Autodesk Inventor part; units mm, degrees
(part 5 of 6)
sketch "Block3" plane through (0, 0, 0) normal (0, 0, 1) x (1, 0, 0)
  arc A0 (-2.9788, 59.5057) -> (-3.9405, 59.975) centre (-5.1609, 56.2539) ccw
  arc A1 (-3.9405, 59.975) -> (-4.1922, 59.6845) centre (0, 56.3062) ccw
  arc A2 (-3.5908, 58.7994) -> (-3.7596, 58.5369) centre (0, 56.3062) ccw
  arc A3 (-3.7596, 58.5369) -> (-4.8145, 58.7162) centre (-4.9371, 54.802) ccw
  arc A4 (-4.8145, 58.7162) -> (-4.9742, 58.3666) centre (0, 56.3062) ccw
  arc A5 (-4.1478, 57.6868) -> (-4.2357, 57.3874) centre (0, 56.3062) ccw
  arc A6 (-4.9742, 58.3666) -> (-4.1478, 57.6868) centre (-2.0963, 61.0225) ccw
  arc A7 (-4.1922, 59.6845) -> (-3.5908, 58.7994) centre (-0.6827, 61.4221) ccw
  arc A8 (-4.1478, 54.9257) -> (-4.9742, 54.2459) centre (-2.0963, 51.59) ccw
  arc A9 (-4.9742, 54.2459) -> (-4.8145, 53.8963) centre (0, 56.3062) ccw
  arc A10 (-4.8145, 53.8963) -> (-3.7596, 54.0756) centre (-4.9371, 57.8105) ccw
  arc A11 (-3.7596, 54.0756) -> (-3.5908, 53.8131) centre (0, 56.3062) ccw
  arc A12 (-3.5908, 53.8131) -> (-4.1922, 52.928) centre (-0.6827, 51.1904) ccw
  arc A13 (-4.1922, 52.928) -> (-3.9405, 52.6375) centre (0, 56.3062) ccw
  arc A14 (-3.9405, 52.6375) -> (-2.9788, 53.1068) centre (-5.1609, 56.3586) ccw
  arc A15 (-2.9788, 53.1068) -> (-2.743, 52.9024) centre (0, 56.3062) ccw
  arc A16 (0.4673, 51.9598) -> (0.7762, 52.0042) centre (0, 56.3062) ccw
  arc A17 (0.1922, 50.9257) -> (0.4673, 51.9598) centre (-3.4193, 52.4401) ccw
  arc A18 (-0.1922, 50.9257) -> (0.1922, 50.9257) centre (0, 56.3062) ccw
  arc A19 (-0.4673, 51.9598) -> (-0.1922, 50.9257) centre (3.4193, 52.4401) ccw
  arc A20 (-0.7762, 52.0042) -> (-0.4673, 51.9598) centre (0, 56.3062) ccw
  arc A21 (-1.3315, 51.0895) -> (-0.7762, 52.0042) centre (-4.37, 53.5601) ccw
  arc A22 (-1.7003, 51.1978) -> (-1.3315, 51.0895) centre (0, 56.3062) ccw
  arc A23 (-1.6729, 52.2675) -> (-1.7003, 51.1978) centre (2.1915, 51.6334) ccw
  arc A24 (-1.9568, 52.3971) -> (-1.6729, 52.2675) centre (0, 56.3062) ccw
  arc A25 (-2.7473, 51.6759) -> (-1.9568, 52.3971) centre (-4.9666, 54.9025) ccw
  arc A26 (-2.743, 52.9024) -> (-3.0706, 51.8837) centre (0.7863, 51.2053) ccw
  arc A27 (-3.0706, 51.8837) -> (-2.7473, 51.6759) centre (0, 56.3062) ccw
  arc A28 (3.7596, 54.0756) -> (4.8145, 53.8963) centre (4.9371, 57.8105) ccw
  arc A29 (4.8145, 53.8963) -> (4.9742, 54.2459) centre (0, 56.3062) ccw
  arc A30 (4.9742, 54.2459) -> (4.1478, 54.9257) centre (2.0963, 51.59) ccw
  arc A31 (4.1478, 54.9257) -> (4.2357, 55.2251) centre (0, 56.3062) ccw
  arc A32 (4.2357, 55.2251) -> (5.2985, 55.3503) centre (4.3134, 59.1405) ccw
  arc A33 (5.2985, 55.3503) -> (5.3532, 55.7307) centre (0, 56.3062) ccw
  arc A34 (4.3687, 56.1502) -> (4.3687, 56.4623) centre (0, 56.3062) ccw
  arc A35 (5.3532, 55.7307) -> (4.3687, 56.1502) centre (3.3401, 52.3716) ccw
  arc A36 (4.3687, 56.4623) -> (5.3532, 56.8818) centre (3.3401, 60.2409) ccw
  arc A37 (5.2985, 57.2622) -> (4.2357, 57.3874) centre (4.3134, 53.472) ccw
  arc A38 (5.3532, 56.8818) -> (5.2985, 57.2622) centre (0, 56.3062) ccw
  arc A39 (3.0706, 60.7288) -> (2.7473, 60.9366) centre (0, 56.3062) ccw
  arc A40 (2.743, 59.7101) -> (3.0706, 60.7288) centre (-0.7863, 61.4072) ccw
  arc A41 (2.9788, 59.5057) -> (2.743, 59.7101) centre (0, 56.3062) ccw
  arc A42 (3.9405, 59.975) -> (2.9788, 59.5057) centre (5.1609, 56.2539) ccw
  arc A43 (4.1922, 59.6845) -> (3.9405, 59.975) centre (0, 56.3062) ccw
  arc A44 (3.7596, 58.5369) -> (3.5908, 58.7994) centre (0, 56.3062) ccw
  arc A45 (3.5908, 58.7994) -> (4.1922, 59.6845) centre (0.6827, 61.4221) ccw
  arc A46 (4.2357, 57.3874) -> (4.1478, 57.6868) centre (0, 56.3062) ccw
  arc A47 (4.9742, 58.3666) -> (4.8145, 58.7162) centre (0, 56.3062) ccw
  arc A48 (4.1478, 57.6868) -> (4.9742, 58.3666) centre (2.0963, 61.0225) ccw
  arc A49 (4.8145, 58.7162) -> (3.7596, 58.5369) centre (4.9371, 54.802) ccw
  arc A50 (-4.2357, 55.2251) -> (-4.1478, 54.9257) centre (0, 56.3062) ccw
  arc A51 (-5.2985, 55.3503) -> (-4.2357, 55.2251) centre (-4.3134, 59.1405) ccw
  arc A52 (-5.3532, 55.7307) -> (-5.2985, 55.3503) centre (0, 56.3062) ccw
  arc A53 (-4.3687, 56.4623) -> (-4.3687, 56.1502) centre (0, 56.3062) ccw
  arc A54 (-4.3687, 56.1502) -> (-5.3532, 55.7307) centre (-3.3401, 52.3716) ccw
  arc A55 (-5.2985, 57.2622) -> (-5.3532, 56.8818) centre (0, 56.3062) ccw
  arc A56 (-4.2357, 57.3874) -> (-5.2985, 57.2622) centre (-4.3134, 53.472) ccw
  arc A57 (-5.3532, 56.8818) -> (-4.3687, 56.4623) centre (-3.3401, 60.2409) ccw
  arc A58 (0.7762, 52.0042) -> (1.3315, 51.0895) centre (4.37, 53.5601) ccw
  arc A59 (1.3315, 51.0895) -> (1.7003, 51.1978) centre (0, 56.3062) ccw
  arc A60 (1.7003, 51.1978) -> (1.6729, 52.2675) centre (-2.1915, 51.6334) ccw
  arc A61 (2.7473, 60.9366) -> (1.9568, 60.2154) centre (4.9666, 57.71) ccw
  arc A62 (1.9568, 60.2154) -> (1.6729, 60.345) centre (0, 56.3062) ccw
  arc A63 (1.6729, 60.345) -> (1.7003, 61.4147) centre (-2.1915, 60.9791) ccw
  arc A64 (1.7003, 61.4147) -> (1.3315, 61.523) centre (0, 56.3062) ccw
  arc A65 (0.7762, 60.6083) -> (0.4673, 60.6527) centre (0, 56.3062) ccw
  arc A66 (1.3315, 61.523) -> (0.7762, 60.6083) centre (4.37, 59.0524) ccw
  arc A67 (-0.4673, 60.6527) -> (-0.7762, 60.6083) centre (0, 56.3062) ccw
  arc A68 (0.1922, 61.6868) -> (-0.1922, 61.6868) centre (0, 56.3062) ccw
  arc A69 (-0.1922, 61.6868) -> (-0.4673, 60.6527) centre (3.4193, 60.1724) ccw
  arc A70 (0.4673, 60.6527) -> (0.1922, 61.6868) centre (-3.4193, 60.1724) ccw
  arc A71 (3.5908, 53.8131) -> (3.7596, 54.0756) centre (0, 56.3062) ccw
  arc A72 (4.1922, 52.928) -> (3.5908, 53.8131) centre (0.6827, 51.1904) ccw
  arc A73 (3.9405, 52.6375) -> (4.1922, 52.928) centre (0, 56.3062) ccw
  arc A74 (2.9788, 53.1068) -> (3.9405, 52.6375) centre (5.1609, 56.3586) ccw
  arc A75 (2.743, 52.9024) -> (2.9788, 53.1068) centre (0, 56.3062) ccw
  arc A76 (1.6729, 52.2675) -> (1.9568, 52.3971) centre (0, 56.3062) ccw
  arc A77 (2.7473, 51.6759) -> (3.0706, 51.8837) centre (0, 56.3062) ccw
  arc A78 (1.9568, 52.3971) -> (2.7473, 51.6759) centre (4.9666, 54.9025) ccw
  arc A79 (3.0706, 51.8837) -> (2.743, 52.9024) centre (-0.7863, 51.2053) ccw
  arc A80 (-2.743, 59.7101) -> (-2.9788, 59.5057) centre (0, 56.3062) ccw
  arc A81 (-3.0706, 60.7288) -> (-2.743, 59.7101) centre (0.7863, 61.4072) ccw
  arc A82 (-2.7473, 60.9366) -> (-3.0706, 60.7288) centre (0, 56.3062) ccw
  arc A83 (-1.6729, 60.345) -> (-1.9568, 60.2154) centre (0, 56.3062) ccw
  arc A84 (-1.9568, 60.2154) -> (-2.7473, 60.9366) centre (-4.9666, 57.71) ccw
  arc A85 (-1.7003, 61.4147) -> (-1.6729, 60.345) centre (2.1915, 60.9791) ccw
  arc A86 (-0.7762, 60.6083) -> (-1.3315, 61.523) centre (-4.37, 59.0524) ccw
  arc A87 (-1.3315, 61.523) -> (-1.7003, 61.4147) centre (0, 56.3062) ccw
  point P0 (-0.0135, 56.3062)
  point P1 (-4.75, 56.3062)
sketch "Sketch1" plane through (0, 0, 0) normal (0, 0, 1) x (1, 0, 0)
  arc A0 (-1.2609, -14.9469) -> (-1.2609, 14.9469) centre (0, 0) ccw
  arc A1 (-8.2391, 14.9469) -> (-8.2391, -14.9469) centre (-9.5, 0) ccw
  line L0 (-9.5, 0) -> (0, 0) construction
  arc A2 (-8.2391, 14.9469) -> (-1.2609, 14.9469) centre (-4.75, 56.3062) ccw
  arc A3 (-1.2609, -14.9469) -> (-8.2391, -14.9469) centre (-4.75, -56.3062) ccw
  circle A4 centre (-4.75, 0) radius 11.5
  line L1 (-24.5, 15) -> (15, 15) construction
  line L2 (15, 15) -> (15, -15) construction
  line L3 (15, -15) -> (-24.5, -15) construction
  line L4 (-24.5, -15) -> (-24.5, 15) construction
  dimension "d0" = 9.5
  dimension "d2" = 15
  dimension "d4" = 23
  dimension "d13" = 39.5
  dimension "d14" = 0.2
  constraints: 10 end point, 8 point on circle, 8 tangent, 5 centre point, 2 equal radius, 2 horizontal, 2 parallel, 1 coincident, 1 midpoint, 1 perpendicular
  measures "d0" distance of L0.start L0.end
  measures "d2" radius of A1
  measures "d4" diameter of A4
  measures "d13" distance between parallel lines of L2 L4
  measures "d14" distance edge to line of A2 L1
extrude "Extrusion1" add sketch "Sketch1" along normal mid plane 11
sketch "Sketch8" plane through (0, 0, 5.5) normal (0, 0, 1) x (1, 0, 0)
  arc A0 (-1.2609, -14.9469) -> (-1.2609, 14.9469) centre (0, 0) ccw construction
  arc A1 (-8.2391, 14.9469) -> (-1.2609, 14.9469) centre (-4.75, 56.3062) ccw construction
  arc A2 (-8.2391, 14.9469) -> (-8.2391, -14.9469) centre (-9.5, 0) ccw construction
  arc A3 (-1.2609, -14.9469) -> (-8.2391, -14.9469) centre (-4.75, -56.3062) ccw construction
  circle A4 centre (-4.75, 0) radius 11.5 construction
  arc A5 (-1.2021, -14.2494) -> (-1.2021, 14.2494) centre (0, 0) ccw
  arc A6 (-1.2021, -14.2494) -> (-8.2979, -14.2494) centre (-4.75, -56.3062) ccw
  arc A7 (-8.2979, 14.2494) -> (-8.2979, -14.2494) centre (-9.5, 0) ccw
  arc A8 (-8.2979, 14.2494) -> (-1.2021, 14.2494) centre (-4.75, 56.3062) ccw
  dimension "d27" = 0.7
  constraints: 8 point on circle, 4 centre point, 3 other
  measures "d27" radial gap between concentric circles of A0 A5
extrude "Extrusion7" cut sketch "Sketch8" against normal blind 0.3
mirror "Mirror1" about plane through (0, 0, 0) normal (0, 0, 1) of "Extrusion7"
chamfer "Chamfer1" distance 0.3 angle 45 8 edges at (14.3, 0, 5.5) (-4.75, -14.1, 5.5) (-23.8, 0, 5.5) (-4.75, 14.1, 5.5) (14.3, 0, -5.5) (-4.75, 14.1, -5.5) (-23.8, 0, -5.5) (-4.75, -14.1, -5.5)
sketch "Sketch12" plane through (-4.75, -56.3062, -5.2) normal (0, 0, -1) x (-1, 0, 0)
  circle A0 centre (0, 56.3062) radius 11.5 projected
  circle A1 centre (0, 56.3062) radius 7.5
  point P0 (-4.75, 56.3062)
  dimension "d42" = 15
  constraints: 1 centre point, 1 coincident
  measures "d42" diameter of A1
extrude "Extrusion11" add sketch "Sketch12" along normal blind 5 and the other way blind 2.5 contours A1
spur gear teeth "Spur Gear1" teeth 24 pitch diameter 9.6 tip diameter 10.251 root diameter 8.451 face width 2 trims to tip circle yes start plane through (-4.75, 0, -10.2) normal (0, 0, -1) x (-1, 0, 0)
sketch "Sketch13" plane through (-4.75, 0, -8.2) normal (0, 0, -1) x (-1, 0, 0)
  arc A0 (2.4162, -4.5203) -> (2.7066, -4.3526) centre (0, 0) ccw projected
  arc A1 (1.7439, -3.8489) -> (2.4162, -4.5203) centre (4.6311, -1.6304) ccw projected
  arc A2 (1.4884, -3.9547) -> (1.7439, -3.8489) centre (0, 0) ccw projected
  arc A3 (1.4879, -4.9048) -> (1.4884, -3.9547) centre (-2.1219, -4.4276) ccw projected
  arc A4 (1.1639, -4.9916) -> (1.4879, -4.9048) centre (0, 0) ccw projected
  arc A5 (0.6883, -4.1691) -> (1.1639, -4.9916) centre (4.0514, -2.7734) ccw projected
  arc A6 (0.4142, -4.2052) -> (0.6883, -4.1691) centre (0, 0) ccw projected
  arc A7 (0.1677, -5.1228) -> (0.4142, -4.2052) centre (-3.1955, -3.7275) ccw projected
  arc A8 (-0.1677, -5.1228) -> (0.1677, -5.1228) centre (0, 0) ccw projected
  arc A9 (-0.4142, -4.2052) -> (-0.1677, -5.1228) centre (3.1955, -3.7275) ccw projected
  arc A10 (-0.6883, -4.1691) -> (-0.4142, -4.2052) centre (0, 0) ccw projected
  arc A11 (-1.1639, -4.9916) -> (-0.6883, -4.1691) centre (-4.0514, -2.7734) ccw projected
  arc A12 (-1.4879, -4.9048) -> (-1.1639, -4.9916) centre (0, 0) ccw projected
  arc A13 (-1.4884, -3.9547) -> (-1.4879, -4.9048) centre (2.1219, -4.4276) ccw projected
  arc A14 (-1.7439, -3.8489) -> (-1.4884, -3.9547) centre (0, 0) ccw projected
  arc A15 (-2.4162, -4.5203) -> (-1.7439, -3.8489) centre (-4.6311, -1.6304) ccw projected
  arc A16 (-2.7066, -4.3526) -> (-2.4162, -4.5203) centre (0, 0) ccw projected
  arc A17 (-2.4613, -3.4347) -> (-2.7066, -4.3526) centre (0.9036, -4.8259) ccw projected
  arc A18 (-2.6806, -3.2664) -> (-2.4613, -3.4347) centre (0, 0) ccw projected
  arc A19 (-3.5038, -3.7409) -> (-2.6806, -3.2664) centre (-4.8953, -0.3762) ccw projected
  arc A20 (-3.7409, -3.5038) -> (-3.5038, -3.7409) centre (0, 0) ccw projected
  arc A21 (-3.2664, -2.6806) -> (-3.7409, -3.5038) centre (-0.3762, -4.8953) ccw projected
  arc A22 (-3.4347, -2.4613) -> (-3.2664, -2.6806) centre (0, 0) ccw projected
  arc A23 (-4.3526, -2.7066) -> (-3.4347, -2.4613) centre (-4.8259, 0.9036) ccw projected
  arc A24 (-4.5203, -2.4162) -> (-4.3526, -2.7066) centre (0, 0) ccw projected
  arc A25 (-3.8489, -1.7439) -> (-4.5203, -2.4162) centre (-1.6304, -4.6311) ccw projected
  arc A26 (-3.9547, -1.4884) -> (-3.8489, -1.7439) centre (0, 0) ccw projected
  arc A27 (-4.9048, -1.4879) -> (-3.9547, -1.4884) centre (-4.4276, 2.1219) ccw projected
  arc A28 (-4.9916, -1.1639) -> (-4.9048, -1.4879) centre (0, 0) ccw projected
  arc A29 (-4.1691, -0.6883) -> (-4.9916, -1.1639) centre (-2.7734, -4.0514) ccw projected
  arc A30 (-4.2052, -0.4142) -> (-4.1691, -0.6883) centre (0, 0) ccw projected
  arc A31 (-5.1228, -0.1677) -> (-4.2052, -0.4142) centre (-3.7275, 3.1955) ccw projected
  arc A32 (-5.1228, 0.1677) -> (-5.1228, -0.1677) centre (0, 0) ccw projected
  arc A33 (-4.2052, 0.4142) -> (-5.1228, 0.1677) centre (-3.7275, -3.1955) ccw projected
  arc A34 (-4.1691, 0.6883) -> (-4.2052, 0.4142) centre (0, 0) ccw projected
  arc A35 (-4.9916, 1.1639) -> (-4.1691, 0.6883) centre (-2.7734, 4.0514) ccw projected
  arc A36 (-4.9048, 1.4879) -> (-4.9916, 1.1639) centre (0, 0) ccw projected
  arc A37 (-3.9547, 1.4884) -> (-4.9048, 1.4879) centre (-4.4276, -2.1219) ccw projected
  arc A38 (-3.8489, 1.7439) -> (-3.9547, 1.4884) centre (0, 0) ccw projected
  arc A39 (-4.5203, 2.4162) -> (-3.8489, 1.7439) centre (-1.6304, 4.6311) ccw projected
  arc A40 (-4.3526, 2.7066) -> (-4.5203, 2.4162) centre (0, 0) ccw projected
  arc A41 (-3.4347, 2.4613) -> (-4.3526, 2.7066) centre (-4.8259, -0.9036) ccw projected
  arc A42 (-3.2664, 2.6806) -> (-3.4347, 2.4613) centre (0, 0) ccw projected
  arc A43 (-3.7409, 3.5038) -> (-3.2664, 2.6806) centre (-0.3762, 4.8953) ccw projected
  arc A44 (-3.5038, 3.7409) -> (-3.7409, 3.5038) centre (0, 0) ccw projected
  arc A45 (-2.6806, 3.2664) -> (-3.5038, 3.7409) centre (-4.8953, 0.3762) ccw projected
  arc A46 (-2.4613, 3.4347) -> (-2.6806, 3.2664) centre (0, 0) ccw projected
  arc A47 (-2.7066, 4.3526) -> (-2.4613, 3.4347) centre (0.9036, 4.8259) ccw projected
  arc A48 (-2.4162, 4.5203) -> (-2.7066, 4.3526) centre (0, 0) ccw projected
  arc A49 (-1.7439, 3.8489) -> (-2.4162, 4.5203) centre (-4.6311, 1.6304) ccw projected
  arc A50 (-1.4884, 3.9547) -> (-1.7439, 3.8489) centre (0, 0) ccw projected
  arc A51 (-1.4879, 4.9048) -> (-1.4884, 3.9547) centre (2.1219, 4.4276) ccw projected
  arc A52 (-1.1639, 4.9916) -> (-1.4879, 4.9048) centre (0, 0) ccw projected
  arc A53 (-0.6883, 4.1691) -> (-1.1639, 4.9916) centre (-4.0514, 2.7734) ccw projected
  arc A54 (-0.4142, 4.2052) -> (-0.6883, 4.1691) centre (0, 0) ccw projected
  arc A55 (-0.1677, 5.1228) -> (-0.4142, 4.2052) centre (3.1955, 3.7275) ccw projected
  arc A56 (0.1677, 5.1228) -> (-0.1677, 5.1228) centre (0, 0) ccw projected
  arc A57 (0.4142, 4.2052) -> (0.1677, 5.1228) centre (-3.1955, 3.7275) ccw projected
  arc A58 (0.6883, 4.1691) -> (0.4142, 4.2052) centre (0, 0) ccw projected
  arc A59 (1.1639, 4.9916) -> (0.6883, 4.1691) centre (4.0514, 2.7734) ccw projected
  arc A60 (1.4879, 4.9048) -> (1.1639, 4.9916) centre (0, 0) ccw projected
  arc A61 (2.6806, -3.2664) -> (3.5038, -3.7409) centre (4.8953, -0.3762) ccw projected
  arc A62 (2.4613, -3.4347) -> (2.6806, -3.2664) centre (0, 0) ccw projected
  arc A63 (2.7066, -4.3526) -> (2.4613, -3.4347) centre (-0.9036, -4.8259) ccw projected
  circle A64 centre (0, 0) radius 7.5 projected
  arc A65 (3.9547, -1.4884) -> (4.9048, -1.4879) centre (4.4276, 2.1219) ccw projected
  arc A66 (3.8489, -1.7439) -> (3.9547, -1.4884) centre (0, 0) ccw projected
  arc A67 (4.5203, -2.4162) -> (3.8489, -1.7439) centre (1.6304, -4.6311) ccw projected
  arc A68 (4.3526, -2.7066) -> (4.5203, -2.4162) centre (0, 0) ccw projected
  arc A69 (3.4347, -2.4613) -> (4.3526, -2.7066) centre (4.8259, 0.9036) ccw projected
  arc A70 (3.2664, -2.6806) -> (3.4347, -2.4613) centre (0, 0) ccw projected
  arc A71 (3.7409, -3.5038) -> (3.2664, -2.6806) centre (0.3762, -4.8953) ccw projected
  arc A72 (3.5038, -3.7409) -> (3.7409, -3.5038) centre (0, 0) ccw projected
  arc A73 (2.7066, 4.3526) -> (2.4162, 4.5203) centre (0, 0) ccw projected
  arc A74 (2.4613, 3.4347) -> (2.7066, 4.3526) centre (-0.9036, 4.8259) ccw projected
  arc A75 (2.6806, 3.2664) -> (2.4613, 3.4347) centre (0, 0) ccw projected
  arc A76 (3.5038, 3.7409) -> (2.6806, 3.2664) centre (4.8953, 0.3762) ccw projected
  arc A77 (3.7409, 3.5038) -> (3.5038, 3.7409) centre (0, 0) ccw projected
  arc A78 (3.2664, 2.6806) -> (3.7409, 3.5038) centre (0.3762, 4.8953) ccw projected
  arc A79 (3.4347, 2.4613) -> (3.2664, 2.6806) centre (0, 0) ccw projected
  arc A80 (4.3526, 2.7066) -> (3.4347, 2.4613) centre (4.8259, -0.9036) ccw projected
  arc A81 (4.5203, 2.4162) -> (4.3526, 2.7066) centre (0, 0) ccw projected
  arc A82 (3.8489, 1.7439) -> (4.5203, 2.4162) centre (1.6304, 4.6311) ccw projected
  arc A83 (3.9547, 1.4884) -> (3.8489, 1.7439) centre (0, 0) ccw projected
  arc A84 (4.9048, 1.4879) -> (3.9547, 1.4884) centre (4.4276, -2.1219) ccw projected
  arc A85 (4.9916, 1.1639) -> (4.9048, 1.4879) centre (0, 0) ccw projected
  arc A86 (4.1691, 0.6883) -> (4.9916, 1.1639) centre (2.7734, 4.0514) ccw projected
  arc A87 (4.2052, 0.4142) -> (4.1691, 0.6883) centre (0, 0) ccw projected
  arc A88 (5.1228, 0.1677) -> (4.2052, 0.4142) centre (3.7275, -3.1955) ccw projected
  arc A89 (5.1228, -0.1677) -> (5.1228, 0.1677) centre (0, 0) ccw projected
  arc A90 (4.2052, -0.4142) -> (5.1228, -0.1677) centre (3.7275, 3.1955) ccw projected
  arc A91 (4.1691, -0.6883) -> (4.2052, -0.4142) centre (0, 0) ccw projected
  arc A92 (4.9916, -1.1639) -> (4.1691, -0.6883) centre (2.7734, -4.0514) ccw projected
  arc A93 (4.9048, -1.4879) -> (4.9916, -1.1639) centre (0, 0) ccw projected
  arc A94 (1.4884, 3.9547) -> (1.4879, 4.9048) centre (-2.1219, 4.4276) ccw projected
  arc A95 (1.7439, 3.8489) -> (1.4884, 3.9547) centre (0, 0) ccw projected
  arc A96 (2.4162, 4.5203) -> (1.7439, 3.8489) centre (4.6311, 1.6304) ccw projected
  point P0 (-4.75, 0)
extrude "Extrusion12" cut sketch "Sketch13" against normal through all
sketch "Sketch14" plane through (-4.75, -56.3062, -10.2) normal (0, 0, -1) x (-1, 0, 0)
  circle A0 centre (0, 56.3062) radius 11.5 projected
  circle A1 centre (0, 56.3062) radius 9.9126
  point P0 (-4.75, 56.3062)
  constraints: 1 centre point, 1 coincident
extrude "Extrusion13" cut sketch "Sketch14" against normal up to surface (5 mm away) contours A1
sketch "Sketch15" plane through (-1.5545, 3.7275, -5.2) normal (0, 0, -1) x (-0.9657677, 0.2594086, 0)
  circle A0 centre (2.1192, -4.4288) radius 11.5 projected
  circle A1 centre (2.1192, -4.4288) radius 3.95
  point P0 (-2.4682, -3.1967)
  dimension "d51" = 7.9
  constraints: 1 centre point, 1 coincident
  measures "d51" diameter of A1
extrude "Extrusion14" cut sketch "Sketch15" against normal through all contours A1
sketch "Sketch16" plane through (-4.75, 0, -5.2) normal (0, 0, -1) x (-0.9659258, -0.258819, 0)
  circle A0 centre (0, 0) radius 11.5 projected
  circle A1 centre (0, 0) radius 4.3255
  arc A2 (-3.2664, -2.6806) -> (-3.7409, -3.5038) centre (-0.3762, -4.8953) ccw projected
  circle A3 centre (0, 0) radius 4.2255
  point P0 (-4.5881, -1.2294)
  dimension "d54" = 0.1
  constraints: 2 coincident, 1 centre point, 3 other
extrude "Extrusion15" add sketch "Sketch16" against normal up to surface (2.5 mm away) contours A1
chamfer "Chamfer2" distance 2 distance2 1 1 edges at (-16.25, 0, -5.2) measured on face at (-16.25, 0, -4.7)
sketch "Sketch17" plane through (-4.75, -56.3062, -2.7) normal (0, 0, 1) x (1, 0, 0)
  circle A0 centre (0, 56.3062) radius 11.5 projected
  circle A1 centre (0, 56.3062) radius 3.95 projected
extrude "Extrusion16" add sketch "Sketch17" along normal blind 1.2
sketch "Sketch19" plane through (0, 0, 5.2) normal (0, 0, 1) x (1, 0, 0)
  circle A0 centre (-4.75, 0) radius 11.5 construction
  circle A1 centre (-4.75, 0) radius 13
  point P0 (0, 0)
  dimension "d67" = 26
  constraints: 1 centre point, 1 coincident
  measures "d67" diameter of A1
extrude "Extrusion17" cut sketch "Sketch19" against normal up to surface (6.7 mm away)
sketch "Sketch18" plane through (0, 0, 0) normal (0, 1, 0) x (-1, 0, 0)
  line L0 (4.75, -1.5) -> (4.75, 10.534) construction
  line L1 (17.75, 5.2) -> (13.3, 5.2)
  line L2 (13.8, 4.7) -> (13.8, 0.4)
  line L3 (13.8, 0.4) -> (13.3, 0.4)
  line L4 (13.3, 0.4) -> (13.3, -1.5)
  line L5 (13.3, -1.5) -> (4.75, -1.5) construction
  line L6 (-6.75, -1.5) -> (16.25, -1.5) construction
  line L7 (13.3, -1.5) -> (16.25, -1.5)
  line L8 (16.25, 5.2) -> (-6.75, 5.2) construction
  line L9 (-8.25, 5.2) -> (17.75, 5.2) construction
  line L10 (17.75, -1.5) -> (17.75, -1.5) construction
  line L11 (17.75, 5.2) -> (17.75, -1.5)
  line L12 (17.75, -1.5) -> (16.25, -1.5)
  line L13 (13.3, 5.2) -> (13.3, 4.7)
  line L14 (13.3, 4.7) -> (13.8, 4.7)
  point P0 (4.75, 5.2)
  dimension "d62" = 9.05
  dimension "d63" = 0.5
  dimension "d64" = 4.3
  dimension "d66" = 1.9
  dimension "d70" = 0
  dimension "d106" = 0.5
  dimension "d107" = 0.5
  constraints: 22 end point, 6 perpendicular, 3 vertical, 2 horizontal, 2 midpoint, 1 point on line
  measures "d62" distance between parallel lines of L0 L2
  measures "d63" distance of L2.end L3.end
  measures "d64" distance of L2.start L2.end
  measures "d66" distance of L3.end L4.end
  measures "d70" distance between parallel lines of L1 L9
  measures "d106" distance of L1.end L13.end
  measures "d107" distance of L13.end L2.start
revolve "Revolution1" add sketch "Sketch18" angle 360 about axis through (-4.75, 0, -1.5) along (0, 0, 1)
ref_plane "Work Plane2" through (0, 0, 0) normal (0, 0, 1) x (1, 0, 0)
sketch "Sketch21" plane through (0, 0, 0) normal (0, 0, 1) x (1, 0, 0)
  circle A0 centre (-4.75, 0) radius 9.05 projected
  line L0 (-4.75, 0) -> (-15.2041, 13.8731) construction
  line L1 (-4.75, 0) -> (-26.3613, 0) construction
  arc A1 (-8.2391, 14.9469) -> (-8.2391, -14.9469) centre (-9.5, 0) ccw construction
  line L2 (-15.2041, 13.8731) -> (-16.4078, 15.4704) construction
  line L3 (-16.4078, 15.4704) -> (-10.7682, 7.9864) construction
  line L4 (-15.2789, 12.7261) -> (-17.0067, 15.019)
  line L5 (-17.0067, 15.019) -> (-15.8088, 15.9217)
  line L6 (-15.8088, 15.9217) -> (-14.081, 13.6288)
  line L7 (-14.081, 13.6288) -> (-15.2789, 12.7261)
  line L8 (-15.2789, 12.7261) -> (-15.8088, 15.9217) construction
  line L9 (-17.0067, 15.019) -> (-14.081, 13.6288) construction
  point P0 (0, 0)
  point P1 (-13.588, 11.7284)
  point P2 (-15.5439, 14.3239)
  dimension "d75" = 53
  dimension "d76" = 2
  dimension "d81" = 16.5
  dimension "d82" = 1.5
  constraints: 22 end point, 4 midpoint, 3 parallel, 2 point on line, 1 collinear, 1 horizontal, 1 perpendicular, 1 point on circle
  measures "d75" angle of L0 L1
  measures "d76" distance of L0.end L2.end
  measures "d81" distance from line of L0.start L7
  measures "d82" distance of L4.end L5.end
extrude "Extrusion19" cut sketch "Sketch21" against normal mid plane 6 contours L4 L5 L6 L7
ref_plane "Work Plane3" through (-12.1194, 8.5333, 3) normal (-0.601815, 0.7986355, 0) x (0.7986355, 0.601815, 0)
sketch "Sketch24" plane through (-12.1194, 8.5333, 3) normal (-0.601815, 0.7986355, 0) x (0.7986355, 0.601815, 0)
  line L0 (0, 6) -> (0, 0) construction
  line L1 (0, 0) -> (1.5, 0) construction
  line L2 (1.5, 0) -> (1.5, 6) construction
  line L3 (1.5, 6) -> (0, 6) construction
  line L4 (-1.25, 7.75) -> (2.75, 7.75)
  line L5 (2.75, 7.75) -> (2.75, 6.25)
  line L6 (2.75, 6.25) -> (-1.25, 6.25)
  line L7 (-1.25, 6.25) -> (-1.25, 7.75)
  line L8 (-1.25, 7.75) -> (2.75, 6.25) construction
  line L9 (2.75, 7.75) -> (-1.25, 6.25) construction
  line L10 (0.75, 7) -> (0.75, 6) construction
  point P0 (4.5435, 3)
  dimension "d99" = 1
  dimension "d100" = 1.5
  dimension "d101" = 4
  constraints: 14 end point, 3 midpoint, 2 parallel, 1 horizontal, 1 perpendicular, 1 vertical
  measures "d99" distance of L10.start L10.end
  measures "d100" distance of L4.end L5.end
  measures "d101" distance of L4.start L4.end
sketch "Sketch25" plane through (-15.2789, 12.7261, 3) normal (-0.601815, 0.7986355, 0) x (0.7986355, 0.601815, 0)
  line L0 (0, 6) -> (0, 0) projected
  line L1 (0, 0) -> (1.5, 0) projected
  line L2 (1.5, 0) -> (1.5, 6) projected
  line L3 (1.5, 6) -> (0, 6) projected
  point P0 (4.5435, 3)
loft "Loft1" cut profiles "Sketch24", "Sketch25"
sketch "Sketch22" plane through (-4.75, 0, 5.2) normal (0, 0, 1) x (1, 0, 0)
  circle A0 centre (-9.5, -5.5) radius 1
  circle A1 centre (0, 0) radius 3.95 projected
  point P0 (4.75, 0)
  dimension "d88" = 5.5
  dimension "d89" = 9.5
  dimension "d90" = 2
  constraints: 1 centre point
  measures "d88" vertical distance of A0.centre A1.centre
  measures "d89" horizontal distance of A1.centre A0.centre
  measures "d90" diameter of A0
extrude "Extrusion20" cut sketch "Sketch22" against normal blind 4 contours A0
sketch "Sketch23" plane through (-14.25, -5.5, 1.2) normal (0, 0, 1) x (1, 0, 0)
  circle A0 centre (0, 0) radius 1 construction
  line L0 (0, 0) -> (-6.6144, -4.5) construction
  line L1 (-0.5625, 0.8268) -> (-7.1769, -3.6732)
  line L2 (-6.0519, -5.3268) -> (0.5625, -0.8268)
  arc A1 (0.5625, -0.8268) -> (-0.5625, 0.8268) centre (0, 0) ccw
  arc A2 (-7.1769, -3.6732) -> (-6.0519, -5.3268) centre (-6.6144, -4.5) ccw
  circle A3 centre (9.5, 5.5) radius 3.95 projected
  point P0 (-3.3072, -2.25)
  dimension "d93" = 10
  dimension "d94" = 8
  constraints: 8 end point, 4 point on circle, 4 tangent, 2 centre point, 1 concentric, 1 midpoint, 1 parallel
  measures "d93" vertical distance of A3.centre L0.end
  measures "d94" distance of L0.start L0.end
extrude "Extrusion21" cut sketch "Sketch23" along normal mid plane 3 contours A1 L2 A2 L1
pattern_circular "Circular Pattern2" count 2 over 360 about axis through (-4.75, 0, -5.2) along (0, 0, 1) of "Extrusion19", "Extrusion20", "Extrusion21", "Loft1"
fillet "Fillet2" radius 1 8 edges at (-20.7468, -9.9252, -0.3) (-21.3883, -9.147, 1.2) (-20.7468, -9.9252, 2.7) (-20.0545, -10.6585, 1.2) (11.2468, 9.9252, 2.7) (11.8883, 9.147, 1.2) (11.2468, 9.9252, -0.3) (10.5545, 10.6585, 1.2)
sketch "Sketch26" plane through (-4.75, -56.3062, -2.7) normal (0, 0, -1) x (-1, 0, 0)
  arc A0 (-5.2349, 46.0668) -> (8.3998, 64.1608) centre (0, 56.3062) ccw projected
  circle A1 centre (0, 56.3062) radius 11.45
  circle A2 centre (0, 56.3062) radius 23.5644
  arc A3 (-5.2349, 46.0668) -> (8.3998, 64.1608) centre (0, 56.3062) ccw projected
  circle A4 centre (0, 56.3062) radius 11.5
  point P0 (-4.75, 56.3062)
  point P1 (8.3998, 64.1608)
  dimension "d108" = 0.05
  constraints: 3 coincident, 2 centre point, 3 other
  measures "d108" radial gap between concentric circles of A0 A1
extrude "Extrusion22" cut sketch "Sketch26" along normal mid plane 36.5 contours A4 A0 | A2
ref_plane "Work Plane4" through (-4.75, -56.3062, -0.9) normal (0, 0, -1) x (-1, 0, 0)
sketch "Sketch27" plane through (-4.75, -56.3062, -0.9) normal (0, 0, -1) x (-1, 0, 0)
  circle A0 centre (0.0119, 55.9035) radius 37.3016
  point P0 (-4.75, 56.3062)
  constraints: 1 centre point
extrude "Extrusion23" cut sketch "Sketch27" against normal through all
sketch "Sketch28" plane through (-4.75, 0, -0.9) normal (0, 0, 1) x (1, 0, 0)
  line L0 (18.7681, 21.7252) -> (10, 21.7252)
  line L1 (10, 21.7252) -> (10, -19.8553)
  line L2 (10, -19.8553) -> (18.7681, -19.8553)
  line L3 (18.7681, -19.8553) -> (18.7681, 21.7252)
  line L4 (-19.6954, 20.4967) -> (-10, 20.4967)
  line L5 (-10, 20.4967) -> (-10, -19.0939)
  line L6 (-10, -19.0939) -> (-19.6954, -19.0939)
  line L7 (-19.6954, -19.0939) -> (-19.6954, 20.4967)
  circle A0 centre (0, 0) radius 3.95 projected
  line L8 (0, 0) -> (0, 16.0604) construction
  point P0 (4.75, 0)
  dimension "d116" = 10
  dimension "d117" = 10
  dimension "d120" = 0
  constraints: 18 end point, 5 parallel, 2 perpendicular, 1 vertical
  measures "d116" distance from line of L8.start L5
  measures "d117" distance from line of L8.start L1
  measures "d120" angle of L8 L1
extrude "Extrusion24" cut sketch "Sketch28" against normal through all contours L3 L2 L1 L0 | L4 L5 L6 L7
sketch "Sketch29" plane through (-4.75, -56.3062, -2.7) normal (0, 0, -1) x (-1, 0, 0)
  line L0 (-10, 61.8832) -> (-10, 50.7293) projected
  line L1 (-10, 56.3062) -> (10, 56.3062)
  line L2 (10, 50.7293) -> (10, 61.8832) projected
  point P0 (-4.75, 56.3062)
  constraints: 2 end point, 2 midpoint
sketch "Sketch30" plane through (-9.1776, 2.1219, -5.2) normal (0, 0, -1) x (-0.9998912, 0.0147508, 0)
  circle A0 centre (-4.4584, -2.0563) radius 3.95 projected
  arc A1 (-0.424, -3.6164) -> (0.424, -3.6164) centre (0, 0) ccw projected
  arc A2 (0.424, -3.6164) -> (0.5155, -3.2937) centre (-4.4584, -2.0563) ccw projected
  arc A3 (0.5155, -3.2937) -> (-0.206, -2.8483) centre (-1.745, -6.1482) ccw projected
  arc A4 (-0.206, -2.8483) -> (-0.1577, -2.5191) centre (-4.4584, -2.0563) ccw projected
  arc A5 (-0.1577, -2.5191) -> (0.6614, -2.2996) centre (-0.6841, 1.0838) ccw projected
  arc A6 (0.6614, -2.2996) -> (0.6663, -1.9642) centre (-4.4584, -2.0563) ccw projected
  arc A7 (0.6663, -1.9642) -> (-0.1459, -1.7207) centre (-0.7784, -5.3065) ccw projected
  arc A8 (-0.1459, -1.7207) -> (-0.1845, -1.3902) centre (-4.4584, -2.0563) ccw projected
  arc A9 (-0.1845, -1.3902) -> (0.5499, -0.9662) centre (-1.6255, 1.9537) ccw projected
  arc A10 (0.5499, -0.9662) -> (0.4679, -0.641) centre (-4.4584, -2.0563) ccw projected
  arc A11 (0.4679, -0.641) -> (-0.3797, -0.616) centre (-0.0626, -4.2433) ccw projected
  arc A12 (-0.3797, -0.616) -> (-0.5025, -0.3067) centre (-4.4584, -2.0563) ccw projected
  arc A13 (-0.5025, -0.3067) -> (0.0971, 0.2929) centre (-2.7599, 2.5503) ccw projected
  arc A14 (0.0971, 0.2929) -> (-0.0663, 0.5858) centre (-4.4584, -2.0563) ccw projected
  arc A15 (-0.0663, 0.5858) -> (-0.8915, 0.3906) centre (0.3536, -3.0311) ccw projected
  arc A16 (-0.8915, 0.3906) -> (-1.0901, 0.6575) centre (-4.4584, -2.0563) ccw projected
  arc A17 (-1.0901, 0.6575) -> (-0.6662, 1.3919) centre (-4.01, 2.8329) ccw projected
  arc A18 (-0.6662, 1.3919) -> (-0.8998, 1.6325) centre (-4.4584, -2.0563) ccw projected
  arc A19 (-0.8998, 1.6325) -> (-1.6463, 1.2304) centre (0.442, -1.7524) ccw projected
  arc A20 (-1.6463, 1.2304) -> (-1.9073, 1.4368) centre (-4.4584, -2.0563) ccw projected
  arc A21 (-1.9073, 1.4368) -> (-1.6878, 2.2559) centre (-5.2907, 2.7823) ccw projected
  arc A22 (-1.6878, 2.2559) -> (-1.9758, 2.4278) centre (-4.4584, -2.0563) ccw projected
  arc A23 (-1.9758, 2.4278) -> (-2.5928, 1.8462) centre (0.1963, -0.4945) ccw projected
  arc A24 (-2.5928, 1.8462) -> (-2.8983, 1.9781) centre (-4.4584, -2.0563) ccw projected
  arc A25 (-2.8983, 1.9781) -> (-2.8983, 2.826) centre (-6.5147, 2.402) ccw projected
  arc A26 (-2.8983, 2.826) -> (-3.221, 2.9176) centre (-4.4584, -2.0563) ccw projected
  arc A27 (-3.221, 2.9176) -> (-3.6664, 2.1961) centre (-0.3665, 0.657) ccw projected
  arc A28 (-3.6664, 2.1961) -> (-3.9957, 2.2444) centre (-4.4584, -2.0563) ccw projected
  arc A29 (-3.9957, 2.2444) -> (-4.2151, 3.0634) centre (-7.5986, 1.7179) ccw projected
  arc A30 (-4.2151, 3.0634) -> (-4.5505, 3.0684) centre (-4.4584, -2.0563) ccw projected
  arc A31 (-4.5505, 3.0684) -> (-4.794, 2.2561) centre (-1.2082, 1.6236) ccw projected
  arc A32 (-4.794, 2.2561) -> (-5.1245, 2.2176) centre (-4.4584, -2.0563) ccw projected
  arc A33 (-5.1245, 2.2176) -> (-5.5485, 2.9519) centre (-8.4684, 0.7766) ccw projected
  arc A34 (-5.5485, 2.9519) -> (-5.8737, 2.8699) centre (-4.4584, -2.0563) ccw projected
  arc A35 (-5.8737, 2.8699) -> (-5.8987, 2.0223) centre (-2.2714, 2.3394) ccw projected
  arc A36 (-5.8987, 2.0223) -> (-6.208, 1.8995) centre (-4.4584, -2.0563) ccw projected
  arc A37 (-6.208, 1.8995) -> (-6.8076, 2.4991) centre (-9.065, -0.3578) ccw projected
  arc A38 (-6.8076, 2.4991) -> (-7.1005, 2.3357) centre (-4.4584, -2.0563) ccw projected
  arc A39 (-7.1005, 2.3357) -> (-6.9053, 1.5106) centre (-3.4836, 2.7557) ccw projected
  arc A40 (-6.9053, 1.5106) -> (-7.1722, 1.3119) centre (-4.4584, -2.0563) ccw projected
  arc A41 (-7.1722, 1.3119) -> (-7.9066, 1.7359) centre (-9.3476, -1.608) ccw projected
  arc A42 (-7.9066, 1.7359) -> (-8.1472, 1.5022) centre (-4.4584, -2.0563) ccw projected
  arc A43 (-8.1472, 1.5022) -> (-7.7451, 0.7557) centre (-4.7623, 2.844) ccw projected
  arc A44 (-7.7451, 0.7557) -> (-7.9515, 0.4947) centre (-4.4584, -2.0563) ccw projected
  arc A45 (-7.9515, 0.4947) -> (-8.7706, 0.7142) centre (-9.297, -2.8887) ccw projected
  arc A46 (-8.7706, 0.7142) -> (-8.9425, 0.4262) centre (-4.4584, -2.0563) ccw projected
  arc A47 (-8.9425, 0.4262) -> (-8.3609, -0.1908) centre (-6.0202, 2.5984) ccw projected
  arc A48 (-8.3609, -0.1908) -> (-8.4928, -0.4963) centre (-4.4584, -2.0563) ccw projected
  arc A49 (-8.4928, -0.4963) -> (-9.3407, -0.4963) centre (-8.9167, -4.1127) ccw projected
  arc A50 (-9.3407, -0.4963) -> (-9.4323, -0.819) centre (-4.4584, -2.0563) ccw projected
  arc A51 (-9.4323, -0.819) -> (-8.7108, -1.2644) centre (-7.1717, 2.0355) ccw projected
  arc A52 (-8.7108, -1.2644) -> (-8.7591, -1.5936) centre (-4.4584, -2.0563) ccw projected
  arc A53 (-8.7591, -1.5936) -> (-9.5781, -1.8131) centre (-8.2326, -5.1965) ccw projected
  arc A54 (-9.5781, -1.8131) -> (-9.5831, -2.1485) centre (-4.4584, -2.0563) ccw projected
  arc A55 (-9.5831, -2.1485) -> (-8.7709, -2.392) centre (-8.1383, 1.1938) ccw projected
  arc A56 (-8.7709, -2.392) -> (-8.7323, -2.7225) centre (-4.4584, -2.0563) ccw projected
  arc A57 (-8.7323, -2.7225) -> (-9.4666, -3.1465) centre (-7.2913, -6.0664) ccw projected
  arc A58 (-9.4666, -3.1465) -> (-9.3846, -3.4717) centre (-4.4584, -2.0563) ccw projected
  arc A59 (-9.3846, -3.4717) -> (-8.537, -3.4967) centre (-8.8541, 0.1306) ccw projected
  arc A60 (-8.537, -3.4967) -> (-8.4142, -3.806) centre (-4.4584, -2.0563) ccw projected
  arc A61 (-8.4142, -3.806) -> (-9.0138, -4.4056) centre (-6.1569, -6.6629) ccw projected
  arc A62 (-9.0138, -4.4056) -> (-8.8504, -4.6985) centre (-4.4584, -2.0563) ccw projected
  arc A63 (-8.8504, -4.6985) -> (-8.0253, -4.5033) centre (-9.2704, -1.0816) ccw projected
  arc A64 (-8.0253, -4.5033) -> (-7.8266, -4.7702) centre (-4.4584, -2.0563) ccw projected
  arc A65 (-7.8266, -4.7702) -> (-8.2506, -5.5045) centre (-4.9067, -6.9456) ccw projected
  arc A66 (-8.2506, -5.5045) -> (-8.0169, -5.7452) centre (-4.4584, -2.0563) ccw projected
  arc A67 (-8.0169, -5.7452) -> (-7.2704, -5.3431) centre (-9.3587, -2.3603) ccw projected
  arc A68 (-7.2704, -5.3431) -> (-7.0094, -5.5495) centre (-4.4584, -2.0563) ccw projected
  arc A69 (-7.0094, -5.5495) -> (-7.2289, -6.3685) centre (-3.626, -6.895) ccw projected
  arc A70 (-7.2289, -6.3685) -> (-6.9409, -6.5405) centre (-4.4584, -2.0563) ccw projected
  arc A71 (-6.9409, -6.5405) -> (-6.3239, -5.9589) centre (-9.1131, -3.6182) ccw projected
  arc A72 (-6.3239, -5.9589) -> (-6.0184, -6.0907) centre (-4.4584, -2.0563) ccw projected
  arc A73 (-6.0184, -6.0907) -> (-6.0184, -6.9387) centre (-2.402, -6.5147) ccw projected
  arc A74 (-6.0184, -6.9387) -> (-5.6958, -7.0303) centre (-4.4584, -2.0563) ccw projected
  arc A75 (-5.6958, -7.0303) -> (-5.2503, -6.3087) centre (-8.5502, -4.7697) ccw projected
  arc A76 (-5.2503, -6.3087) -> (-4.9211, -6.357) centre (-4.4584, -2.0563) ccw projected
  arc A77 (-4.9211, -6.357) -> (-4.7016, -7.1761) centre (-1.3182, -5.8306) ccw projected
  arc A78 (-4.7016, -7.1761) -> (-4.3663, -7.181) centre (-4.4584, -2.0563) ccw projected
  arc A79 (-4.3663, -7.181) -> (-4.1227, -6.3688) centre (-7.7085, -5.7363) ccw projected
  arc A80 (-4.1227, -6.3688) -> (-3.7922, -6.3303) centre (-4.4584, -2.0563) ccw projected
  arc A81 (-3.7922, -6.3303) -> (-3.3682, -7.0646) centre (-0.4483, -4.8892) ccw projected
  arc A82 (-3.3682, -7.0646) -> (-3.043, -6.9826) centre (-4.4584, -2.0563) ccw projected
  arc A83 (-3.043, -6.9826) -> (-3.018, -6.135) centre (-6.6453, -6.4521) ccw projected
  arc A84 (-3.018, -6.135) -> (-2.7087, -6.0122) centre (-4.4584, -2.0563) ccw projected
  arc A85 (-2.7087, -6.0122) -> (-2.1092, -6.6118) centre (0.1482, -3.7548) ccw projected
  arc A86 (-2.1092, -6.6118) -> (-1.8162, -6.4484) centre (-4.4584, -2.0563) ccw projected
  arc A87 (-1.8162, -6.4484) -> (-2.0115, -5.6232) centre (-5.4331, -6.8684) ccw projected
  arc A88 (-2.0115, -5.6232) -> (-1.7445, -5.4246) centre (-4.4584, -2.0563) ccw projected
  arc A89 (-1.7445, -5.4246) -> (-1.0102, -5.8486) centre (0.4309, -2.5047) ccw projected
  arc A90 (-1.0102, -5.8486) -> (-0.7695, -5.6149) centre (-4.4584, -2.0563) ccw projected
  arc A91 (-0.7695, -5.6149) -> (-1.1716, -4.8684) centre (-4.1544, -6.9567) ccw projected
  arc A92 (-1.1716, -4.8684) -> (-0.9652, -4.6074) centre (-4.4584, -2.0563) ccw projected
  arc A93 (-0.9652, -4.6074) -> (-0.1462, -4.8269) centre (0.3803, -1.224) ccw projected
  arc A94 (-0.1462, -4.8269) -> (0.0258, -4.5389) centre (-4.4584, -2.0563) ccw projected
  arc A95 (0.0258, -4.5389) -> (-0.5558, -3.9219) centre (-2.8965, -6.711) ccw projected
  arc A96 (-0.5558, -3.9219) -> (-0.424, -3.6164) centre (-4.4584, -2.0563) ccw projected
  arc A97 (-7.1711, 1.2484) -> (-7.8968, 1.6771) centre (-9.3476, -1.608) ccw
  arc A98 (-6.8448, 1.4912) -> (-7.1711, 1.2484) centre (-4.4584, -2.0563) ccw
  arc A99 (-7.047, 2.3094) -> (-6.8448, 1.4912) centre (-3.4836, 2.7557) ccw
  arc A100 (-6.8134, 2.4398) -> (-7.047, 2.3094) centre (-4.4584, -2.0563) ccw
  arc A101 (-6.2233, 1.8379) -> (-6.8134, 2.4398) centre (-9.065, -0.3578) ccw
  arc A102 (-5.8453, 1.988) -> (-6.2233, 1.8379) centre (-4.4584, -2.0563) ccw
  arc A103 (-5.8288, 2.8307) -> (-5.8453, 1.988) centre (-2.2714, 2.3394) ccw
  arc A104 (-5.5694, 2.8961) -> (-5.8288, 2.8307) centre (-4.4584, -2.0563) ccw
  arc A105 (-5.1553, 2.162) -> (-5.5694, 2.8961) centre (-8.4684, 0.7766) ccw
  arc A106 (-4.7513, 2.2091) -> (-5.1553, 2.162) centre (-4.4584, -2.0563) ccw
  arc A107 (-4.5173, 3.0188) -> (-4.7513, 2.2091) centre (-1.2082, 1.6236) ccw
  arc A108 (-4.2498, 3.0149) -> (-4.5173, 3.0188) centre (-4.4584, -2.0563) ccw
  arc A109 (-4.0397, 2.1986) -> (-4.2498, 3.0149) centre (-7.5986, 1.7179) ccw
  arc A110 (-3.6374, 2.1396) -> (-4.0397, 2.1986) centre (-4.4584, -2.0563) ccw
  arc A111 (-3.2017, 2.8612) -> (-3.6374, 2.1396) centre (-0.3665, 0.657) ccw
  arc A112 (-2.9444, 2.7881) -> (-3.2017, 2.8612) centre (-4.4584, -2.0563) ccw
  arc A113 (-2.9527, 1.9453) -> (-2.9444, 2.7881) centre (-6.5147, 2.402) ccw
  arc A114 (-2.5793, 1.7841) -> (-2.9527, 1.9453) centre (-4.4584, -2.0563) ccw
  arc A115 (-1.9718, 2.3683) -> (-2.5793, 1.7841) centre (0.1963, -0.4945) ccw
  arc A116 (-1.7421, 2.2312) -> (-1.9718, 2.3683) centre (-4.4584, -2.0563) ccw
  arc A117 (-1.9683, 1.4193) -> (-1.7421, 2.2312) centre (-5.2907, 2.7823) ccw
  arc A118 (-1.6494, 1.167) -> (-1.9683, 1.4193) centre (-4.4584, -2.0563) ccw
  arc A119 (-0.9113, 1.574) -> (-1.6494, 1.167) centre (0.442, -1.7524) ccw
  arc A120 (-0.725, 1.3821) -> (-0.9113, 1.574) centre (-4.4584, -2.0563) ccw
  arc A121 (-1.1536, 0.6564) -> (-0.725, 1.3821) centre (-4.01, 2.8329) ccw
  arc A122 (-0.9108, 0.3301) -> (-1.1536, 0.6564) centre (-4.4584, -2.0563) ccw
  arc A123 (-0.0926, 0.5323) -> (-0.9108, 0.3301) centre (0.3536, -3.0311) ccw
  arc A124 (0.0377, 0.2986) -> (-0.0926, 0.5323) centre (-4.4584, -2.0563) ccw
  arc A125 (-0.5641, -0.2914) -> (0.0377, 0.2986) centre (-2.7599, 2.5503) ccw
  arc A126 (-0.4141, -0.6694) -> (-0.5641, -0.2914) centre (-4.4584, -2.0563) ccw
  arc A127 (0.4286, -0.6859) -> (-0.4141, -0.6694) centre (-0.0626, -4.2433) ccw
  arc A128 (0.4941, -0.9453) -> (0.4286, -0.6859) centre (-4.4584, -2.0563) ccw
  arc A129 (-0.24, -1.3595) -> (0.4941, -0.9453) centre (-1.6255, 1.9537) ccw
  arc A130 (-0.1929, -1.7634) -> (-0.24, -1.3595) centre (-4.4584, -2.0563) ccw
  arc A131 (0.6168, -1.9974) -> (-0.1929, -1.7634) centre (-0.7784, -5.3065) ccw
  arc A132 (0.6129, -2.2649) -> (0.6168, -1.9974) centre (-4.4584, -2.0563) ccw
  arc A133 (-0.2034, -2.475) -> (0.6129, -2.2649) centre (-0.6841, 1.0838) ccw
  arc A134 (-0.2624, -2.8774) -> (-0.2034, -2.475) centre (-4.4584, -2.0563) ccw
  arc A135 (0.4591, -3.313) -> (-0.2624, -2.8774) centre (-1.745, -6.1482) ccw
  arc A136 (0.3861, -3.5703) -> (0.4591, -3.313) centre (-4.4584, -2.0563) ccw
  arc A137 (-0.4567, -3.562) -> (0.3861, -3.5703) centre (0, 0) ccw
  arc A138 (-0.6179, -3.9354) -> (-0.4567, -3.562) centre (-4.4584, -2.0563) ccw
  arc A139 (-0.0337, -4.5429) -> (-0.6179, -3.9354) centre (-2.8965, -6.711) ccw
  arc A140 (-0.1708, -4.7726) -> (-0.0337, -4.5429) centre (-4.4584, -2.0563) ccw
  arc A141 (-0.9828, -4.5464) -> (-0.1708, -4.7726) centre (0.3803, -1.224) ccw
  arc A142 (-1.2351, -4.8653) -> (-0.9828, -4.5464) centre (-4.4584, -2.0563) ccw
  arc A143 (-0.828, -5.6034) -> (-1.2351, -4.8653) centre (-4.1544, -6.9567) ccw
  arc A144 (-1.02, -5.7897) -> (-0.828, -5.6034) centre (-4.4584, -2.0563) ccw
  arc A145 (-1.7457, -5.3611) -> (-1.02, -5.7897) centre (0.4309, -2.5047) ccw
  arc A146 (-2.0719, -5.6039) -> (-1.7457, -5.3611) centre (-4.4584, -2.0563) ccw
  arc A147 (-1.8698, -6.4221) -> (-2.0719, -5.6039) centre (-5.4331, -6.8684) ccw
  arc A148 (-2.1034, -6.5524) -> (-1.8698, -6.4221) centre (-4.4584, -2.0563) ccw
  arc A149 (-2.6934, -5.9506) -> (-2.1034, -6.5524) centre (0.1482, -3.7548) ccw
  arc A150 (-3.0714, -6.1007) -> (-2.6934, -5.9506) centre (-4.4584, -2.0563) ccw
  arc A151 (-3.0879, -6.9433) -> (-3.0714, -6.1007) centre (-6.6453, -6.4521) ccw
  arc A152 (-3.3473, -7.0088) -> (-3.0879, -6.9433) centre (-4.4584, -2.0563) ccw
  arc A153 (-3.7615, -6.2747) -> (-3.3473, -7.0088) centre (-0.4483, -4.8892) ccw
  arc A154 (-4.1654, -6.3218) -> (-3.7615, -6.2747) centre (-4.4584, -2.0563) ccw
  arc A155 (-4.3995, -7.1315) -> (-4.1654, -6.3218) centre (-7.7085, -5.7363) ccw
  arc A156 (-4.6669, -7.1276) -> (-4.3995, -7.1315) centre (-4.4584, -2.0563) ccw
  arc A157 (-4.877, -6.3113) -> (-4.6669, -7.1276) centre (-1.3182, -5.8306) ccw
  arc A158 (-5.2794, -6.2523) -> (-4.877, -6.3113) centre (-4.4584, -2.0563) ccw
  arc A159 (-5.715, -6.9738) -> (-5.2794, -6.2523) centre (-8.5502, -4.7697) ccw
  arc A160 (-5.9724, -6.9008) -> (-5.715, -6.9738) centre (-4.4584, -2.0563) ccw
  arc A161 (-5.964, -6.058) -> (-5.9724, -6.9008) centre (-2.402, -6.5147) ccw
  arc A162 (-6.3374, -5.8968) -> (-5.964, -6.058) centre (-4.4584, -2.0563) ccw
  arc A163 (-6.945, -6.481) -> (-6.3374, -5.8968) centre (-9.1131, -3.6182) ccw
  arc A164 (-7.1746, -6.3439) -> (-6.945, -6.481) centre (-4.4584, -2.0563) ccw
  arc A165 (-6.9484, -5.5319) -> (-7.1746, -6.3439) centre (-3.626, -6.895) ccw
  arc A166 (-7.2674, -5.2796) -> (-6.9484, -5.5319) centre (-4.4584, -2.0563) ccw
  arc A167 (-8.0054, -5.6867) -> (-7.2674, -5.2796) centre (-9.3587, -2.3603) ccw
  arc A168 (-8.1918, -5.4948) -> (-8.0054, -5.6867) centre (-4.4584, -2.0563) ccw
  arc A169 (-7.7631, -4.769) -> (-8.1918, -5.4948) centre (-4.9067, -6.9456) ccw
  arc A170 (-8.0059, -4.4428) -> (-7.7631, -4.769) centre (-4.4584, -2.0563) ccw
  arc A171 (-8.8242, -4.6449) -> (-8.0059, -4.4428) centre (-9.2704, -1.0816) ccw
  arc A172 (-8.9545, -4.4113) -> (-8.8242, -4.6449) centre (-4.4584, -2.0563) ccw
  arc A173 (-8.3526, -3.8213) -> (-8.9545, -4.4113) centre (-6.1569, -6.6629) ccw
  arc A174 (-8.5027, -3.4433) -> (-8.3526, -3.8213) centre (-4.4584, -2.0563) ccw
  arc A175 (-9.3454, -3.4268) -> (-8.5027, -3.4433) centre (-8.8541, 0.1306) ccw
  arc A176 (-9.4108, -3.1674) -> (-9.3454, -3.4268) centre (-4.4584, -2.0563) ccw
  arc A177 (-8.6767, -2.7532) -> (-9.4108, -3.1674) centre (-7.2913, -6.0664) ccw
  arc A178 (-8.7238, -2.3493) -> (-8.6767, -2.7532) centre (-4.4584, -2.0563) ccw
  arc A179 (-9.5336, -2.1152) -> (-8.7238, -2.3493) centre (-8.1383, 1.1938) ccw
  arc A180 (-9.5296, -1.8478) -> (-9.5336, -2.1152) centre (-4.4584, -2.0563) ccw
  arc A181 (-8.7133, -1.6377) -> (-9.5296, -1.8478) centre (-8.2326, -5.1965) ccw
  arc A182 (-8.6543, -1.2353) -> (-8.7133, -1.6377) centre (-4.4584, -2.0563) ccw
  arc A183 (-9.3759, -0.7997) -> (-8.6543, -1.2353) centre (-7.1717, 2.0355) ccw
  arc A184 (-9.3028, -0.5423) -> (-9.3759, -0.7997) centre (-4.4584, -2.0563) ccw
  arc A185 (-8.46, -0.5507) -> (-9.3028, -0.5423) centre (-8.9167, -4.1127) ccw
  arc A186 (-8.2989, -0.1773) -> (-8.46, -0.5507) centre (-4.4584, -2.0563) ccw
  arc A187 (-8.8831, 0.4302) -> (-8.2989, -0.1773) centre (-6.0202, 2.5984) ccw
  arc A188 (-8.7459, 0.6599) -> (-8.8831, 0.4302) centre (-4.4584, -2.0563) ccw
  arc A189 (-7.934, 0.4337) -> (-8.7459, 0.6599) centre (-9.297, -2.8887) ccw
  arc A190 (-7.6817, 0.7527) -> (-7.934, 0.4337) centre (-4.4584, -2.0563) ccw
  arc A191 (-8.0887, 1.4907) -> (-7.6817, 0.7527) centre (-4.7623, 2.844) ccw
  arc A192 (-7.8968, 1.6771) -> (-8.0887, 1.4907) centre (-4.4584, -2.0563) ccw
  point P0 (-9.2079, -1.9863)
  dimension "d121" = 0.05
  constraints: 192 point on circle, 96 centre point, 95 other
  measures "d121" radial gap between concentric circles of A42 A192
extrude "Extrusion25" [suppressed]
sketch "Sketch31" plane through (-4.75, 0, -1.5) normal (0, 0, 1) x (1, 0, 0)
  circle A0 centre (0, 0) radius 8.55 projected
  circle A1 centre (0, 0) radius 3.95 projected
  point P0 (4.75, 0)
extrude "Extrusion26" cut sketch "Sketch31" against normal blind 0.3
fillet "Fillet3" radius 0.2 2 edges at (-0.9352, -1.0247, -5.2) (-8.7, 0, -1.8)
fillet "Fillet4" radius 0.25 8 edges at (-4.75, -11.45, -2.7) (-14.75, 0, -2.7) (-4.75, 11.45, -0.9) (-4.75, 11.45, -2.7) (-4.75, -11.45, -0.9) (-14.75, 0, -0.9) (5.25, 0, -2.7) (5.25, 0, -0.9)
fillet "Fillet4" radius 1 4 edges at (5.25, -5.577, -1.8) (-14.75, -5.577, -1.8) (-14.75, 5.577, -1.8) (5.25, 5.577, -1.8)
sketch "Sketch32" plane through (5.25, -5.3106, -1.15) normal (1, 0, 0) x (0, 0, -1)
  line L0 (0.65, 9.4606) -> (0.65, 1.1606) construction
  circle A0 centre (0.65, 8.2661) radius 0.3155
  circle A1 centre (0.65, 2.106) radius 0.3487
  point P0 (-1.15, 5.3106)
  constraints: 2 centre point, 2 point on line
extrude "Extrusion27" cut sketch "Sketch32" against normal blind 0.2
sketch "Sketch34" plane through (-4.75, -56.3062, -2.7) normal (0, 0, -1) x (-1, 0, 0)
  circle A0 centre (0, 56.3062) radius 4.15 projected
  circle A1 centre (0, 56.3062) radius 6.3266
  point P0 (-4.75, 56.3062)
  constraints: 1 centre point, 1 coincident
extrude "Extrusion28" cut sketch "Sketch34" along normal through all contours A0 | A1